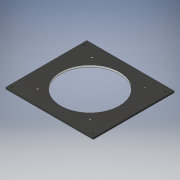
# Autodesk Inventor part: Base Cover Right 6010 Fan
Saved by Autodesk Inventor 2019 (Build 230136000, 136)
## iProperties
Created: 2018-11-05
Part Number: Base Cover Right 6010 Fan
Material: Generic
Document SubType Name: Modeling
Designer: Keith
Density: 1 g/cm^3
Appearance: Default
Author: Keith
## iProperties of the stored document Base Cover Right_3DPrint.ipt
Created: 2018-11-08
Part Number: Base Cover Right_3DPrint
Material: Generic
Document SubType Name: Modeling
Designer: Keith
Density: 1 g/cm^3
Appearance: Default
Author: Keith
Autodesk Inventor part; units mm, degrees
ref_plane "YZ Plane" through (0, 0, 0) normal (1, 0, 0) x (0, 1, 0)
ref_plane "XZ Plane" through (0, 0, 0) normal (0, 1, 0) x (-1, 0, 0)
sketch "Sketch1" plane through (0, 0, 0) normal (0, 1, 0) x (-1, 0, 0)
  line L0 (0, 0) -> (119, 0)
  line L1 (119, 0) -> (119, -110.3)
  line L2 (119, -110.3) -> (0, -110.3)
  line L3 (0, -110.3) -> (0, 0)
  dimension "d0" = 119
  dimension "d1" = 110.3
  constraints: 8 end point, 2 parallel, 1 horizontal, 1 perpendicular
  measures "d0" distance of L1.end L2.end
  measures "d1" distance of L0.end L1.end
extrude "Extrusion1" add sketch "Sketch1" along normal blind 2.5
sketch "Sketch2" plane through (0, 2.5, 0) normal (0, 1, 0) x (1, 0, 0)
  line L0 (-119, 0) -> (0, 0) projected
  line L1 (0, 0) -> (0, 110.3) projected
  line L2 (0, 110.3) -> (-119, 110.3) projected
  line L3 (-119, 110.3) -> (-119, 0) projected
  circle A0 centre (-114.875, 4.375) radius 1.55
  circle A1 centre (-114.875, 103.3) radius 1.55
  dimension "d4" = 3.1
  dimension "d5" = 4.125
  dimension "d6" = 4.375
  dimension "d7" = 3.1
  dimension "d8" = 7
  constraints: 2 centre point
  measures "d4" diameter of A0
  measures "d5" distance from line of L3 A0.centre
  measures "d6" distance from line of L0 A0.centre
  measures "d7" diameter of A1
  measures "d8" distance from line of L2 A1.centre
extrude "Extrusion2" cut sketch "Sketch2" against normal blind 2.5 contours A0 | A1
ref_plane "Work Plane1" through (-59.5, 0, 0) normal (1, 0, 0) x (0, 0, -1)
mirror "Mirror1" about plane through (-59.5, 0, 0) normal (1, 0, 0) of "Extrusion2"
sketch "Sketch3" plane through (0, 2.5, 0) normal (0, 1, 0) x (1, 0, 0)
  circle A0 centre (-4.125, 4.375) radius 1.55 projected
  circle A1 centre (-4.125, 103.3) radius 1.55 projected
  circle A2 centre (-114.875, 4.375) radius 1.55 projected
  circle A3 centre (-114.875, 103.3) radius 1.55 projected
  line L0 (-119, 0) -> (0, 0) projected
  line L1 (0, 0) -> (0, 110.3) projected
  line L2 (0, 110.3) -> (-119, 110.3) projected
  line L3 (-119, 110.3) -> (-119, 0) projected
  circle A4 centre (-59.5, 55.15) radius 40
  circle A5 centre (-23.75, 19.4) radius 1.35
  circle A6 centre (-95.25, 19.4) radius 1.35
  circle A7 centre (-95.25, 93.6) radius 1.35
  circle A8 centre (-23.75, 93.6) radius 1.35
  dimension "d16" = 2.7
  dimension "d17" = 2.7
  dimension "d18" = 2.7
  dimension "d19" = 2.7
  dimension "d30" = 71.5
  dimension "d31" = 71.5
  dimension "d32" = 71.5
  dimension "d34" = 35.75
  dimension "d35" = 35.75
  dimension "d36" = 35.75
  constraints: 5 centre point, 1 other
  measures "d16" diameter of A5
  measures "d17" diameter of A6
  measures "d18" diameter of A7
  measures "d19" diameter of A8
  measures "d30" distance of A8.centre A7.centre
  measures "d32" distance of A6.centre A5.centre
  measures "d34" horizontal distance of A4.centre A6.centre
  measures "d35" horizontal distance of A4.centre A5.centre
  measures "d36" horizontal distance of A4.centre A6.centre
extrude "Extrusion3" cut sketch "Sketch3" against normal blind 2.5 contours A4 | A5 | A6 | A7 | A8
body "Solid1"
